Autodesk Inventor part; units mm, degrees
(part 2 of 2)
ref_plane "Work Plane1" through (-5, 81.9, -49.5) normal (0, 0, -1) x (0, 1, 0)
ref_plane "Work Plane2" through (-13.7357, 64.9938, -40) normal (-0.0348995, 0.9993908, 0) x (-0.9993908, -0.0348995, 0)
ref_plane "Work Plane3" through (-23.8, 0, -27.5) normal (0, 0, -1) x (0, 1, 0)
sketch "Sketch5" plane through (-13.7357, 64.9938, -40) normal (-0.0348995, 0.9993908, 0) x (-0.9993908, -0.0348995, 0)
  arc A0 (0, -0.2709) -> (0, -0.7291) centre (-5.245, -0.5) ccw projected
  arc A1 (0, -0.7291) -> (0, -0.2709) centre (5.245, -0.5) ccw projected
  circle A2 centre (-5.245, -0.5) radius 4.5 projected
  circle A3 centre (5.245, -0.5) radius 4.5 projected
  line L0 (0.5, 1.7467) -> (-0.5, 1.7467)
  line L1 (0.5, -2.7467) -> (-0.5, -2.7467)
  line L2 (0.5, 1.7467) -> (1.346, 1.7467)
  line L3 (-0.5, 1.7467) -> (-1.346, 1.7467)
  line L4 (-0.5, -2.7467) -> (-1.346, -2.7467)
  line L5 (0.5, -2.7467) -> (1.346, -2.7467)
  point P0 (-11.4591, 40)
  dimension "d30" = 1
  dimension "d31" = 1
  constraints: 12 end point, 8 point on circle, 3 point on line, 2 parallel, 1 horizontal
  measures "d30" distance of L0.start L0.end
  measures "d31" distance of L1.start L1.end
extrude "Extrusion14" cut sketch "Sketch5" along normal blind 2.5
extrude "Extrusion15" cut sketch "Sketch5" along normal through all contours A1 L2 A3 L5 A0 L4 A2 L3 | A0 L0 A1 | A0 A1 L1 | A2 | A3
sketch "Sketch8" plane through (-3, 81.4, 35.5) normal (0, 1, 0) x (1, 0, 0)
  line L0 (1.37, 84.5) -> (1.37, 68.5) projected
  line L1 (0.37, 84.5) -> (1.37, 84.5) projected
  line L2 (0.37, 68.5) -> (0.37, 84.5) projected
  line L3 (0.37, 68.5) -> (1.37, 68.5) projected
  line L4 (1.37, 84.5) -> (1.87, 84.5)
  line L5 (1.87, 84.5) -> (1.87, 68)
  line L6 (1.87, 68) -> (0.37, 68)
  line L7 (0.37, 68) -> (0.37, 68.5)
  point P0 (3, 35.5)
  dimension "d54" = 0.5
  dimension "d55" = 0.5
  constraints: 8 end point, 2 perpendicular, 1 horizontal, 1 parallel
  measures "d54" distance between parallel lines of L6 L3
  measures "d55" distance between parallel lines of L5 L0
extrude "Extrusion11" cut sketch "Sketch8" against normal through all
sketch "Sketch9" plane through (-27, 69.2958, -35.5) normal (-1, 0, 0) x (0, 0, 1)
  line L0 (-13.5, -3.7958) -> (2.5, -3.7958) projected
  line L1 (2.5, -3.7958) -> (2.5, 12.2042) projected
  line L2 (2.5, 12.2042) -> (-13.5, 12.2042) projected
  line L3 (-13.5, 12.2042) -> (-13.5, -3.7958) projected
  circle A0 centre (-11.475, 0.3442) radius 0.45 projected
  circle A1 centre (-3, 2.7042) radius 1.25 projected
  circle A2 centre (-11.475, 7.9642) radius 0.45 projected
  circle A3 centre (-11.475, 2.9642) radius 0.45 projected
  circle A4 centre (-11.475, 5.4242) radius 0.45 projected
  line L4 (-10.25, -2.986) -> (-10.25, 17.8025) construction
  line L5 (-13.5, 12.1042) -> (-13.5, -3.9142) projected
  line L6 (-13.5, 8.4142) -> (-11.025, 8.4142)
  line L7 (-11.025, 8.4142) -> (-11.025, -0.1058)
  line L8 (-11.025, -0.1058) -> (-13.5, -0.1058)
  line L9 (-13.5, -0.1058) -> (-13.5, 8.4142)
  ellipse E0 centre (-5, -2.6199) end of major axis (0.25, -2.6199) minor radius 0.1832 (-4.7709, -2.803) -> (-5.2291, -2.803) ccw projected
  ellipse E1 centre (-5, -2.986) end of major axis (0.25, -2.986) minor radius 0.1832 (-5.2291, -2.803) -> (-4.7709, -2.803) ccw projected
  ellipse E2 centre (-5, -2.6199) end of major axis (-0.5, -2.6199) minor radius 0.157 projected
  ellipse E3 centre (-5, -2.986) end of major axis (-0.5, -2.986) minor radius 0.157 projected
  point P0 (35.5, -69.2958)
  point P1 (-16, -3.9142)
  point P2 (-13.5, 8.4142)
  point P3 (-13.5, -0.1058)
  point P4 (-13.5, -3.9142)
  dimension "d58" = 0
  dimension "d59" = 0.775
  dimension "d60" = 0
  dimension "d61" = 0
  constraints: 10 end point, 2 parallel, 2 vertical, 1 horizontal, 1 perpendicular, 5 other
  measures "d58" distance edge to line of A2 L7
  measures "d59" distance between parallel lines of L4 L7
  measures "d60" distance edge to line of A2 L6
  measures "d61" distance edge to line of A0 L8
extrude "Extrusion12" cut sketch "Sketch9" against normal up to surface (25.87 mm away) contours A3 | A4 | L3 L6 A2 L7 A0 L8 | A0 | A0 L7 L8 | L6 L7 A2 | A2
fillet "Fillet1" radius 2 3 edges at (-2.63, 73.45, -46.525) (-2.63, 77.71, -47.7625) (-2.63, 69.19, -47.7625)
sketch "Sketch10" plane through (0, 65.2958, 35.5) normal (1, 0, 0) x (0, 0, -1)
  line L0 (68.5, 16.2042) -> (68.5, 0.2042) projected
  line L1 (68.5, 0.2042) -> (84.5, 0.2042) projected
  line L2 (84.5, 0.2042) -> (84.5, 16.2042) projected
  line L3 (84.5, 16.2042) -> (68.5, 16.2042) projected
  line L4 (80.9, 13.1042) -> (80.9, 9.6042) projected
  line L5 (80.9, 9.6042) -> (77.4, 9.6042) projected
  line L6 (77.4, 9.6042) -> (77.4, 13.1042) projected
  line L7 (77.4, 13.1042) -> (80.9, 13.1042) projected
  line L8 (77.4, 6.8042) -> (80.9, 6.8042) projected
  line L9 (80.9, 6.8042) -> (80.9, 3.3042) projected
  line L10 (80.9, 3.3042) -> (77.4, 3.3042) projected
  line L11 (77.4, 3.3042) -> (77.4, 6.8042) projected
  circle A0 centre (82.475, 4.3442) radius 0.45 projected
  circle A1 centre (74, 6.7042) radius 1.25 projected
  circle A2 centre (82.475, 11.9642) radius 0.45 projected
  circle A3 centre (82.475, 6.9642) radius 0.45 projected
  circle A4 centre (82.475, 9.4242) radius 0.45 projected
  line L12 (76.4, 14.1042) -> (81.9, 14.1042)
  line L13 (81.9, 14.1042) -> (81.9, 2.3042)
  line L14 (81.9, 2.3042) -> (76.4, 2.3042)
  line L15 (76.4, 2.3042) -> (76.4, 14.1042)
  line L16 (76.4, 14.1042) -> (76.4, 16.2042)
  line L17 (81.9, 16.2042) -> (81.9, 14.1042)
  point P0 (35.5, -65.2958)
  dimension "d65" = 1
  dimension "d66" = 1
  dimension "d67" = 1
  dimension "d68" = 1
  constraints: 12 end point, 2 parallel, 2 perpendicular, 2 point on line, 1 collinear, 1 horizontal
  measures "d65" distance between parallel lines of L15 L6
  measures "d66" distance between parallel lines of L12 L7
  measures "d67" distance between parallel lines of L13 L4
  measures "d68" distance between parallel lines of L14 L10
extrude "Extrusion13" cut sketch "Sketch10" against normal up to surface (1.13 mm away) contours L3 L17 L12 L16 | L12 L13 L14 L15 | L4 L5 L6 L7 | L8 L9 L10 L11
ref_plane "Work Plane6" through (-13.7357, 64.9938, -40) normal (-0.0348995, 0.9993908, 0) x (-0.9993908, -0.0348995, 0)
sketch "Sketch12" plane through (-13.7357, 64.9938, -40) normal (-0.0348995, 0.9993908, 0) x (-0.9993908, -0.0348995, 0)
  circle A0 centre (9.6, 6.0491) radius 0.75 projected
  circle A1 centre (0, -6.5) radius 0.75 projected
  circle A2 centre (-9.6, 6.0491) radius 0.75 projected
  point P0 (-11.4591, 40)
hole "Hole2" at (-23.3298, 64.6588, -33.9509) at (-13.7357, 64.9938, -46.5) at (-4.1415, 65.3288, -33.9509) direction (-0.0348995, 0.9993908, 0) diameter 2.5 depth 5 counterbore diameter 3 counterbore depth 1
sketch "Sketch16" plane through (-27, 69.2958, -35.5) normal (-1, 0, 0) x (0, 0, 1)
  line L0 (-11.025, 8.4142) -> (-11.025, -0.1058) projected
  line L1 (-11.025, -0.1058) -> (-13.5, -0.1058) projected
  line L2 (-13.5, -0.1058) -> (-13.5, 8.4142) projected
  line L3 (-13.5, 8.4142) -> (-11.025, 8.4142) projected
  line L4 (-11.025, 8.4142) -> (-11.025, -0.1058) projected
  line L5 (0, 0) -> (0, 17) projected
  line L6 (0, 17) -> (-14.5, 17) projected
  line L7 (-14.5, -4) -> (-14.5, 17) projected
  line L8 (5, -4) -> (-14.5, -4) projected
  line L9 (5, -4) -> (5, 0) projected
  line L10 (0, 0) -> (5, 0) projected
  line L11 (-11.025, 8.4142) -> (0, 8.5)
  line L12 (-12.25, -0.1058) -> (-11.025, -0.1058) projected
  line L13 (-0.5, -1.6205) -> (-0.5, 17.8274) projected
  line L14 (-11.025, -0.1058) -> (0, 0)
  point P0 (35.5, -69.2958)
  point P1 (-0.5, -0.0048)
  point P2 (-0.5, 8.4961)
  constraints: 4 end point, 1 midpoint
extrude "Extrusion16" cut sketch "Sketch16" against normal blind 2 contours L11 L13 L14 L0 | L11 L5 L14 L13
sketch "Sketch15" plane through (-27, 86.2958, -35.5) normal (-0.0465915, 0.998914, 0) x (0.998914, 0.0465915, 0)
  ellipse E0 centre (17.759, 5) end of major axis (13.2587, 5) minor radius 4.5 (13.8597, 2.7533) -> (19.3168, 0.7782) ccw projected
  line L0 (13.8597, 2.7533) -> (11.1676, 2.7533) projected
  ellipse E1 centre (7.2683, 5) end of major axis (2.768, 5) minor radius 4.5 (11.1676, 7.2467) -> (11.1676, 2.7533) ccw projected
  line L1 (11.1676, 7.2467) -> (13.8597, 7.2467) projected
  ellipse E2 centre (17.759, 5) end of major axis (13.2587, 5) minor radius 4.5 (19.3168, 9.2218) -> (13.8597, 7.2467) ccw projected
  line L2 (19.3168, 9.2218) -> (19.3168, 14.5) projected
  line L3 (0, 14.5) -> (19.3168, 14.5) projected
  line L4 (0, 0) -> (0, 14.5) projected
  line L5 (0, 0) -> (19.3168, 0) projected
  line L6 (19.3168, 0) -> (19.3168, 0.7782) projected
  circle A0 centre (12.5137, 11.5) radius 3
  circle A1 centre (3.5265, 11.5) radius 3
  line L7 (0, 14.5) -> (19.3168, 14.5) projected
  line L8 (0, 0) -> (0, 14.5) projected
  ellipse E3 centre (7.2683, 5) end of major axis (2.768, 5) minor radius 4.5 (11.1676, 7.2467) -> (11.1676, 2.7533) ccw projected
  point P0 (22.95, -35.5)
  dimension "d94" = 6
  dimension "d95" = 6
  dimension "d96" = 5.2454
  dimension "d97" = 5.2454
  constraints: 2 centre point, 2 tangent, 5 other
  measures "d94" diameter of A0
  measures "d95" diameter of A1
  measures "d96" horizontal distance of point (7.268, 5) A0.centre
  measures "d97" horizontal distance of A0.centre point (17.759, 5)
hole "Hole3" at (-23.4773, 86.4601, -47) at (-14.4999, 86.8789, -47) direction (0.0465915, -0.998914, 0) diameter 4 depth 4 counterbore diameter 4.5 counterbore depth 0.5
sketch "Sketch17" plane through (-27, 65.2958, -50) normal (-1, 0, 0) x (0, 0, 1)
  line L0 (3.475, 12.4142) -> (14.5, 12.5) projected
  line L1 (14.5, 12.5) -> (14.5, 21) projected
  line L2 (14.5, 21) -> (0, 21) projected
  line L3 (0, 0) -> (0, 21) projected
  line L4 (19.5, 0) -> (0, 0) projected
  line L5 (19.5, 0) -> (19.5, 4) projected
  line L6 (14.5, 4) -> (19.5, 4) projected
  line L7 (14.5, 4) -> (3.475, 3.8942) projected
  line L8 (3.475, 3.8942) -> (1, 3.8942) projected
  line L9 (1, 3.8942) -> (1, 12.4142) projected
  line L10 (1, 12.4142) -> (3.475, 12.4142) projected
  line L11 (0, 12.4494) -> (8, 12.4494)
  line L12 (8, 12.4494) -> (8, 17.4494)
  line L13 (8, 17.4494) -> (0, 17.4494)
  line L14 (0, 17.4494) -> (0, 12.4494)
  line L15 (3.475, 12.4142) -> (14.5, 12.5) projected
  line L16 (8, 17.4494) -> (0, 12.4494)
  line L17 (0, 17.4494) -> (8, 12.4494)
  point P0 (50, -65.2958)
  point P1 (4, 14.9494)
  dimension "d107" = 8
  dimension "d108" = 5
  constraints: 12 end point, 2 parallel, 2 point on line, 1 horizontal, 1 midpoint, 1 perpendicular
  measures "d107" distance of L12.end L13.end
  measures "d108" distance of L11.end L12.end
hole "Hole4" at (-27, 80.2452, -46) direction (1, 0, 0) diameter 4 depth 4.5 counterbore diameter 4.5 counterbore depth 0.5
ref_plane "Work Plane7" through (-13.7357, 64.9938, -40) normal (-0.0348995, 0.9993908, 0) x (-0.9993908, -0.0348995, 0)
sketch "Sketch18" plane through (-13.7357, 64.9938, -40) normal (-0.0348995, 0.9993908, 0) x (-0.9993908, -0.0348995, 0)
  circle A0 centre (0, -6.5) radius 0.75 projected
  circle A1 centre (9.6, 6.0491) radius 0.75 projected
  circle A2 centre (-9.6, 6.0491) radius 0.75 projected
  line L0 (-12.325, 5.5) -> (-12.325, -4.5) projected
  arc A3 (-12.325, -4.5) -> (-8.325, -8.5) centre (-8.325, -4.5) ccw projected
  line L1 (-8.325, -8.5) -> (8.325, -8.5) projected
  arc A4 (8.325, -8.5) -> (12.325, -4.5) centre (8.325, -4.5) ccw projected
  line L2 (12.325, -4.5) -> (12.325, 5.5) projected
  arc A5 (12.325, 5.5) -> (9.325, 8.5) centre (9.325, 5.5) ccw projected
  line L3 (9.325, 8.5) -> (-9.325, 8.5) projected
  arc A6 (-9.325, 8.5) -> (-12.325, 5.5) centre (-9.325, 5.5) ccw projected
  arc A7 (0, -0.2709) -> (0, -0.7291) centre (-5.245, -0.5) ccw projected
  arc A8 (0, -0.7291) -> (0, -0.2709) centre (5.245, -0.5) ccw projected
  line L4 (4.825, 8.5) -> (-4.825, 8.5)
  line L5 (-4.825, 8.5) -> (-4.825, 7)
  line L6 (-4.825, 7) -> (4.825, 7)
  line L7 (4.825, 7) -> (4.825, 8.5)
  line L8 (-13.7379, 9.8) -> (-10.24, 9.8) projected
  line L9 (4.825, 8.5) -> (4.825, 9.8)
  line L10 (-4.825, 8.5) -> (-4.825, 9.8)
  line L11 (-4.825, 9.8) -> (4.825, 9.8)
  point P0 (-11.4591, 40)
  point P1 (-4.825, 8.5)
  point P2 (-4.825, 8.5)
  dimension "d116" = 7.5
  dimension "d117" = 7.5
  dimension "d118" = 1.5
  constraints: 14 end point, 3 perpendicular, 3 point on line, 2 parallel, 1 horizontal, 1 vertical
  measures "d116" distance between parallel lines of L7 L2
  measures "d117" distance between parallel lines of L5 L0
  measures "d118" distance between parallel lines of L4 L6
extrude "Extrusion17" cut sketch "Sketch18" along normal through all contours L10 L11 L9 L3 | L3 L7 L6 L5
sketch "Sketch19" plane through (-23.8, 69.2958, -18.4) normal (0, 1, 0) x (1, 0, 0)
  circle A0 centre (4, 4.55) radius 2.25 projected
  circle A1 centre (4, 4.55) radius 3.5
  line L0 (5.0862, 14.6) -> (14.742, 14.6) projected
  ellipse E0 centre (0.3082, 15.5509) end of major axis (-0.9425, 15.5509) minor radius 1.25 projected
  line L1 (14.5915, 0) -> (14.5915, -37.4) projected
  line L2 (14.5915, -37.4) -> (0, -37.4) projected
  line L3 (0, -37.4) -> (0, -53.9) projected
  line L4 (17.8, -53.9) -> (0, -53.9) projected
  line L5 (17.8, -53.9) -> (17.8, 17.1) projected
  line L6 (-1.2, 17.1) -> (17.8, 17.1) projected
  line L7 (-3.2, 17.1) -> (-1.2, 17.1) projected
  line L8 (-3.2, 17.1) -> (-3.2, 12.1) projected
  line L9 (-3.2, 12.1) -> (0, 12.1) projected
  line L10 (0, 0) -> (0, 12.1) projected
  line L11 (0, 0) -> (14.5915, 0) projected
  line L12 (5.0862, 11.8) -> (0, 6.1)
  line L13 (5.0862, 14.6) -> (0, 12.1)
  line L14 (6.0862, 11.8) -> (6.0862, 14.6)
  line L15 (14.742, 14.6) -> (14.742, 11.8) projected
  line L16 (14.742, 11.8) -> (5.0862, 11.8) projected
  line L17 (5.0862, 11.8) -> (5.0862, 14.6) projected
  point P0 (23.8, -18.4)
  dimension "d121" = 7
  dimension "d122" = 6
  constraints: 6 end point, 2 point on line, 1 centre point, 1 coincident, 1 perpendicular, 1 other
  measures "d121" diameter of A1
  measures "d122" distance of L9.end L12.end
extrude "Extrusion18" cut sketch "Sketch19" against normal blind 2 contours L17 L12 L10 L13 | L0 L14 L16 L17 | L0 L15 L16 L14
mirror "Mirror2" about plane through (0, 0, 0) normal (0, 0, 1) of "Extrusion7", "Extrusion8", "Extrusion9", "Extrusion14", "Extrusion15", "Extrusion11", "Extrusion12", "Fillet1", "Extrusion13", "Hole2", "Extrusion16", "Hole3", "Hole4", "Extrusion17", "Extrusion18"
sketch "Sketch20" plane through (-3, 81.4, -50) normal (1, 0, 0) x (0, 0, -1)
  line L0 (-99.5, 0.5) -> (-99.5, 13.5) projected
  line L1 (-99.5, 0.5) -> (-78, 0.5) projected
  circle A0 centre (-78, 4) radius 3.5 projected
  line L2 (-78, 0.5) -> (-64, 0.5) projected
  circle A1 centre (-64, 4) radius 3.5 projected
  line L3 (-64, 0.5) -> (-50, 0.5) projected
  circle A2 centre (-50, 4) radius 3.5 projected
  line L4 (-50, 0.5) -> (-36, 0.5) projected
  circle A3 centre (-36, 4) radius 3.5 projected
  line L5 (-36, 0.5) -> (-22, 0.5) projected
  circle A4 centre (-22, 4) radius 3.5 projected
  line L6 (-22, 0.5) -> (-0.5, 0.5) projected
  line L7 (-0.5, 13.5) -> (-0.5, 0.5) projected
  line L8 (-99.5, 13.5) -> (-0.5, 13.5) projected
  point P0 (-50, -81.4)
  constraints: 5 vertical alignment
hole "Hole5" at (-3, 85.4, 28) at (-3, 85.4, 14) at (-3, 85.4, 0) at (-3, 85.4, -14) at (-3, 85.4, -28) direction (-1, 0, 0) diameter 2.459 depth 8.8 countersink diameter 3.5 countersink angle 90 thread size "M3x0.5" class "6H" standard "ISO Metric profile"
sketch "Sketch22" plane through (-23.8, 69.2958, -18.4) normal (0, 1, 0) x (1, 0, 0)
  circle A0 centre (14.3, -43.65) radius 2 projected
  circle A1 centre (14.3, -43.65) radius 2.25 projected
  circle A2 centre (4.1, 4.55) radius 2 projected
  circle A3 centre (7.1, -43.65) radius 2 projected
  circle A4 centre (11.3, 4.55) radius 2 projected
  point P0 (23.8, -18.4)
  point P1 (12.7, 4.55)
hole "Hole6" at (-16.7, 69.2958, 25.25) at (-9.5, 69.2958, 25.25) at (-19.7, 69.2958, -22.95) direction (0, -1, 0) diameter 3.4 depth 8.8 countersink diameter 7 countersink angle 90 clearance for "Countersunk Flat Head Screw ISO 2009/7046" size "M3" standard "ISO"
body "Solid2"
